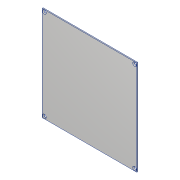
# Autodesk Inventor part: front
Saved by Autodesk Inventor 2017 (Build 210142000, 142)
## iProperties
Created: 2015-10-13
Part Number: front
Material: Aluminum 6061
Document SubType Name: Modeling
Designer: Sawaiz
Density: 2.7 g/cm^3
Appearance: Aluminum - Flat
Mass: 83.3876 g
Surface Area: 398.955 cm^2
Volume: 30.8843 cm^3
Author: Sawaiz
Autodesk Inventor part; units mm, degrees
ref_plane "YZ Plane" through (0, 0, 0) normal (1, 0, 0) x (0, 1, 0)
ref_plane "XZ Plane" through (0, 0, 0) normal (0, 1, 0) x (-1, 0, 0)
ref_plane "XY Plane" through (0, 0, 0) normal (0, 0, 1) x (1, 0, 0)
sketch "Sketch1" plane through (0, 0, 0) normal (1, 0, 0) x (0, 1, 0)
  line L0 (-69.85, -69.85) -> (69.85, -69.85)
  line L1 (69.85, -69.85) -> (69.85, 69.85)
  line L2 (69.85, 69.85) -> (-69.85, 69.85)
  line L3 (-69.85, 69.85) -> (-69.85, -69.85)
  line L4 (-69.85, -69.85) -> (69.85, 69.85) construction
  line L5 (69.85, -69.85) -> (-69.85, 69.85) construction
  point P0 (0, 0)
  dimension "d0" = 139.7
  dimension "d1" = 139.7
  constraints: 12 end point, 2 midpoint, 2 parallel, 1 horizontal, 1 perpendicular
  measures "d0" distance of L2.end L1.end
  measures "d1" distance of L1.end L0.end
extrude "Extrusion1" add sketch "Sketch1" along normal blind 1.5875
sketch "Sketch6" plane through (1.5875, 0, 0) normal (1, 0, 0) x (0, 0, -1)
  line L0 (69.85, -69.85) -> (69.85, 69.85) projected
  line L1 (69.85, 69.85) -> (-69.85, 69.85) projected
  line L2 (-69.85, 69.85) -> (-69.85, -69.85) projected
  line L3 (-69.85, -69.85) -> (69.85, -69.85) projected
  point P0 (0, 0)
  point P1 (-66.675, -66.675)
  dimension "d45" = 3.175
  dimension "d46" = 3.175
  measures "d45" distance from line of L2 point (-66.675, -66.675)
  measures "d46" distance from line of L3 point (-66.675, -66.675)
hole "Hole4" at (1.5875, -66.675, 66.675) direction (-1, 0, 0) diameter 3.2766 end through all countersink diameter 5.715 countersink angle 82 clearance for "Flat Head Machine Screw (82)" size "#4" standard "Ansi Unified Screw Threads"
pattern_circular "Circular Pattern1" count 4 over 360 about axis through (-10, 0, 0) along (1, 0, 0) of "Hole4"
equation "\"d0\" = width + 2 * plasticThickness"
equation "\"d1\" = height + 2 * plasticThickness"
equation "\"d2\" = frontPanelThickness"
equation "\"d45\" = 0.5 * plasticThickness"
equation "\"d46\" = 0.5 * plasticThickness"
equation "\"height\" = 127"
equation "\"width\" = 127"
equation "\"plasticThickness\" = 6.35"
equation "\"caseThickness\" = 6.35"
equation "\"alignmentGrooveDepth\" = 1.5875"
equation "\"alignmentGrooveClearance\" = 0.1016"
equation "\"aerogelHolderDepth\" = 36.5125"
equation "\"depth\" = 190.5"
equation "\"mirrorAngle\" = 5deg"
equation "\"mirrorThickness\" = 3.175"
equation "\"fresnelThickness\" = 0.254"
equation "\"focalLength\" = 152.4"
equation "\"ior\" = 1.49"
equation "\"centerThickness\" = 1.27"
equation "\"fresnelAngle\" = 90deg"
equation "\"fresnelEffectiveDiameter\" = 152.4"
equation "\"frontPanelThickness\" = 1.5875"
body "Solid1"
